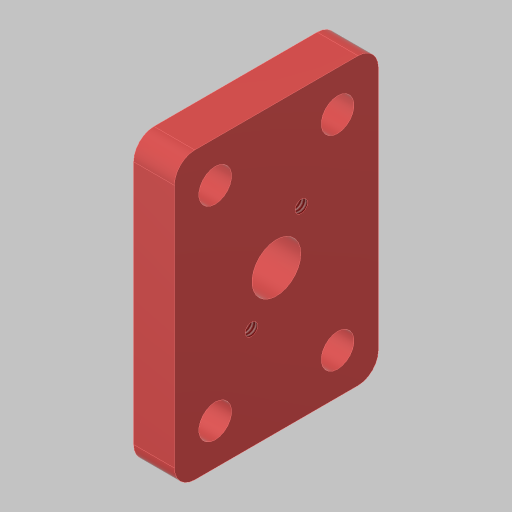
# Autodesk Inventor part: GP5-012
Saved by Autodesk Inventor 2023.5 (Build 275446000, 446)
## iProperties
Created: 2025-02-01
Part Number: GP5-012
Material: ABS Plastic
Document SubType Name: Modeling
Designer: slick
Density: 1.06 g/cm^3
Appearance: Smooth - Red
Author: slick
Autodesk Inventor part; units mm, degrees
ref_plane "YZ Plane" through (0, 0, 0) normal (1, 0, 0) x (0, 1, 0)
ref_plane "XZ Plane" through (0, 0, 0) normal (0, 1, 0) x (-1, 0, 0)
ref_plane "XY Plane" through (0, 0, 0) normal (0, 0, 1) x (1, 0, 0)
sketch "Sketch1" plane through (0, 0, 0) normal (1, 0, 0) x (0, 1, 0)
  line L0 (22.225, 15.875) -> (-22.225, 15.875)
  line L1 (-22.225, 15.875) -> (-22.225, -15.875)
  line L2 (-22.225, -15.875) -> (22.225, -15.875)
  line L3 (22.225, -15.875) -> (22.225, 15.875)
  line L4 (22.225, 15.875) -> (-22.225, -15.875) construction
  line L5 (-22.225, 15.875) -> (22.225, -15.875) construction
  line L6 (15.875, 9.525) -> (-15.875, 9.525) construction
  line L7 (-15.875, 9.525) -> (-15.875, -9.525) construction
  line L8 (-15.875, -9.525) -> (15.875, -9.525) construction
  line L9 (15.875, -9.525) -> (15.875, 9.525) construction
  line L10 (15.875, 9.525) -> (-15.875, -9.525) construction
  line L11 (-15.875, 9.525) -> (15.875, -9.525) construction
  point P0 (0, 0)
  dimension "d0" = 44.45
  dimension "d1" = 31.75
  dimension "d2" = 31.75
  dimension "d3" = 19.05
  constraints: 24 end point, 4 coincident, 4 midpoint, 4 parallel, 2 horizontal, 2 perpendicular
  measures "d0" distance of L2.end L1.end
  measures "d1" distance of L0.end L1.end
  measures "d2" distance of L8.end L7.end
  measures "d3" distance of L7.end L6.end
extrude "Extrusion1" add sketch "Sketch1" along normal blind 6.35
hole "Hole1" at (0, 15.875, 9.525) at (0, 15.875, -9.525) at (0, -15.875, 9.525) at (0, -15.875, -9.525) direction (1, 0, 0) diameter 5.1054 end through all clearance for "Flat Head Machine Screw (82)" size "#10" standard "Ansi Unified Screw Threads"
sketch "Sketch2" plane through (6.35, 0, 0) normal (1, 0, 0) x (0, 0, -1)
  line L0 (3.8812, 6.35) -> (-3.8812, -6.35) construction
  point P0 (0, 0)
  point P1 (0, 0)
  dimension "d13" = 14.8844
  dimension "d27" = 6.35
  constraints: 2 coincident, 2 end point, 1 midpoint
  measures "d13" distance of L0.start L0.end
  measures "d27" vertical distance of L0.start point (0, 0)
hole "Hole2" at (6.35, 6.35, -3.8812) at (6.35, -6.35, 3.8812) direction (-1, 0, 0) diameter 1.9406 end through all thread size "3-48 UNC" class "2B" standard "ANSI Unified Screw Threads"
sketch "Sketch3" plane through (6.35, 0, 0) normal (1, 0, 0) x (0, 0, -1)
  circle A0 centre (0, 0) radius 3.81
  dimension "d21" = 7.62
  constraints: 1 centre point, 1 coincident
  measures "d21" diameter of A0
extrude "Extrusion2" cut sketch "Sketch3" against normal blind 6.35
fillet "Fillet1" radius 3.175 4 edges at (3.175, 22.225, 15.875) (3.175, 22.225, -15.875) (3.175, -22.225, -15.875) (3.175, -22.225, 15.875)
body "Solid1"
